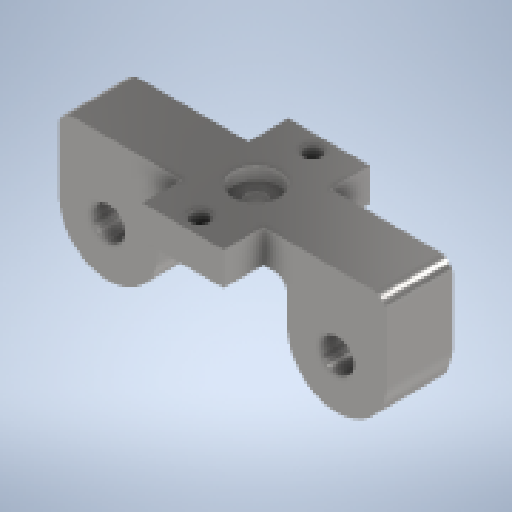
# Autodesk Inventor part: Podstawa chwytaka
Saved by Autodesk Inventor 2024.1 (Build 281209000, 209)
## iProperties
Created: 2024-05-12
Part Number: Podstawa chwytaka
Material: Stal, węglowa
Document SubType Name: Modeling
Designer: Krzysiu
Density: 7.85 g/cm^3
Appearance: Częściowo polerowany
Stock Number: 01
Mass: 49.8719 g
Surface Area: 34.4845 cm^2
Volume: 6.35311 cm^3
Author: Krzysiu
Autodesk Inventor part; units mm, degrees
ref_plane "YZ Plane" through (0, 0, 0) normal (1, 0, 0) x (0, 1, 0)
ref_plane "XZ Plane" through (0, 0, 0) normal (0, 1, 0) x (-1, 0, 0)
ref_plane "XY Plane" through (0, 0, 0) normal (0, 0, 1) x (1, 0, 0)
sketch "Szkic1" plane through (0, 0, 0) normal (0, 0, 1) x (1, 0, 0)
  line L0 (-2.5, 0) -> (-27.5, 0)
  line L1 (-27.5, 0) -> (-19.7354, -28.9778)
  line L2 (-27.5, 0) -> (2.5, 0) construction
  line L3 (-27.5, 0) -> (-37.3351, 36.7052)
  line L4 (-27.5, 0) -> (10.5, 0) construction
  line L5 (-37.3351, 36.7052) -> (-37.3351, 54.7052)
  line L6 (-37.3351, 54.7052) -> (-2.5, 54.7052)
  line L7 (-37.3351, 54.7052) -> (-27.3351, 72.0257)
  line L8 (-37.3351, 54.7052) -> (-17.3351, 54.7052) construction
  line L9 (-37.3351, 54.7052) -> (-27.3351, 37.3847)
  line L10 (-37.3351, 54.7052) -> (-17.3351, 54.7052) construction
  circle A0 centre (-27.5, 0) radius 1.5
  line L11 (-2.5, 0) -> (-2.5, -12)
  line L12 (-2.5, -12) -> (-27.5, -12)
  line L13 (-27.5, -12) -> (-19.7354, -28.9778)
  line L14 (-27.5, -12) -> (-48.0171, 32.862)
  line L15 (-48.0171, 32.862) -> (-51.0127, 50.611)
  line L16 (-48.0171, 32.862) -> (-30.0171, 32.862) construction
  line L17 (-51.0127, 50.611) -> (-38.2696, 35.1962)
  line L18 (-51.0127, 50.611) -> (-31.0127, 50.611) construction
  line L19 (-51.0127, 50.611) -> (-44.0347, 69.3542)
  line L20 (-51.0127, 50.611) -> (-31.0127, 50.611) construction
  circle A1 centre (-27.5, -12) radius 1.5
  line L21 (-19.7354, -28.9778) -> (0, -28.9778)
  circle A2 centre (-19.7354, -28.9778) radius 2.5
  line L22 (-22.2354, -28.9778) -> (-27.2354, -28.9778)
  line L23 (17.2354, -28.9778) -> (22.2354, -28.9778)
  circle A3 centre (14.7354, -28.9778) radius 2.5
  line L24 (22.5, -12) -> (14.7354, -28.9778)
  line L25 (14.7354, -28.9778) -> (0, -28.9778)
  line L26 (-2.5, -12) -> (22.5, -12)
  line L27 (32.3351, 54.7052) -> (22.3351, 37.3847)
  line L28 (32.3351, 36.7052) -> (32.3351, 54.7052)
  line L29 (46.0127, 50.611) -> (33.2696, 35.1962)
  line L30 (43.0171, 32.862) -> (46.0127, 50.611)
  line L31 (43.0171, 32.862) -> (25.0171, 32.862) construction
  circle A4 centre (22.5, 0) radius 1.5
  line L32 (22.5, 0) -> (32.3351, 36.7052)
  circle A5 centre (22.5, -12) radius 1.5
  line L33 (22.5, -12) -> (43.0171, 32.862)
  line L34 (-2.5, 0) -> (22.5, 0)
  line L35 (22.5, 0) -> (14.7354, -28.9778)
  line L36 (22.5, 0) -> (-7.5, 0) construction
  line L37 (22.5, 0) -> (-15.5, 0) construction
  line L38 (46.0127, 50.611) -> (26.0127, 50.611) construction
  line L39 (46.0127, 50.611) -> (26.0127, 50.611) construction
  line L40 (32.3351, 54.7052) -> (12.3351, 54.7052) construction
  line L41 (32.3351, 54.7052) -> (12.3351, 54.7052) construction
  line L42 (32.3351, 54.7052) -> (-2.5, 54.7052)
  line L43 (46.0127, 50.611) -> (39.0347, 69.3542)
  line L44 (32.3351, 54.7052) -> (22.3351, 72.0257)
  line L45 (-19.7354, -31.4778) -> (-19.7354, -36.4778)
  line L46 (-19.7354, -36.4778) -> (0, -36.4778)
  line L47 (-19.7354, -36.4778) -> (-22.2354, -36.4778)
  line L48 (-27.2354, -28.9778) -> (-27.2354, -31.4778)
  line L49 (-19.7354, -26.4778) -> (-19.7354, -21.4778)
  line L50 (-19.7354, -21.4778) -> (-22.2354, -21.4778)
  line L51 (-27.2354, -26.4778) -> (-27.2354, -28.9778)
  line L52 (-19.7354, -21.4778) -> (0, -21.4778)
  line L53 (22.5, 0) -> (14.7354, -28.9778)
  line L54 (22.5, -12) -> (14.7354, -28.9778)
  line L55 (14.7354, -28.9778) -> (-5, -28.9778)
  circle A6 centre (14.7354, -28.9778) radius 2.5
  line L56 (17.2354, -28.9778) -> (22.2354, -28.9778)
  line L57 (-19.7354, -28.9778) -> (-5, -28.9778)
  line L58 (14.7354, -31.4778) -> (14.7354, -36.4778)
  line L59 (14.7354, -36.4778) -> (-5, -36.4778)
  line L60 (14.7354, -36.4778) -> (17.2354, -36.4778)
  line L61 (22.2354, -28.9778) -> (22.2354, -31.4778)
  line L62 (14.7354, -26.4778) -> (14.7354, -21.4778)
  line L63 (14.7354, -21.4778) -> (17.2354, -21.4778)
  line L64 (22.2354, -26.4778) -> (22.2354, -28.9778)
  line L65 (14.7354, -21.4778) -> (-5, -21.4778)
  arc A7 (-22.2354, -21.4778) -> (-27.2354, -26.4778) centre (-22.2354, -26.4778) ccw
  arc A8 (-27.2354, -31.4778) -> (-22.2354, -36.4778) centre (-22.2354, -31.4778) ccw
  arc A9 (22.2354, -26.4778) -> (17.2354, -21.4778) centre (17.2354, -26.4778) ccw
  arc A10 (17.2354, -36.4778) -> (22.2354, -31.4778) centre (17.2354, -31.4778) ccw
  point P0 (0, 0)
  point P1 (-27.2354, -36.4778)
  point P2 (-27.2354, -21.4778)
  point P3 (22.2354, -36.4778)
  point P4 (22.2354, -21.4778)
  dimension "d0" = 25
  dimension "d1" = 30
  dimension "d2" = 75
  dimension "d3" = 38
  dimension "d4" = 105
  dimension "d5" = 18
  dimension "d6" = 20
  dimension "d7" = 60
  dimension "d8" = 20
  dimension "d9" = 60
  dimension "d10" = 3
  dimension "d11" = 12
  dimension "d12" = 25
  dimension "d13" = 49.331
  dimension "d14" = 18
  dimension "d15" = 99.58
  dimension "d16" = 20
  dimension "d17" = 50.42
  dimension "d18" = 20
  dimension "d19" = 69.58
  dimension "d20" = 3
  dimension "d22" = 5
  dimension "d23" = 5
  dimension "d28" = 5
  dimension "d29" = 5
  dimension "d30" = 5
  dimension "d31" = 5
  dimension "d32" = 5
  dimension "d33" = 5
  constraints: 132 end point, 37 symmetric about line, 14 point on circle, 12 horizontal, 12 point on line, 10 centre point, 10 coincident, 8 tangent, 7 equal length, 7 perpendicular, 2 vertical, 1 horizontal alignment, 6 other
  measures "d0" distance of L0.start L0.end
  measures "d1" distance of L0.end L1.end
  measures "d2" angle of L1 L2
  measures "d3" distance of L0.end L3.end
  measures "d4" angle of L4 L3
  measures "d5" distance of L3.end L5.end
  measures "d6" distance of L5.end L7.end
  measures "d7" angle of L8 L7
  measures "d8" distance of L5.end L9.end
  measures "d9" angle of L9 L10
  measures "d10" diameter of A0
  measures "d11" distance of L0.start L11.end
  measures "d12" distance of L11.end L12.end
  measures "d13" distance of L12.end L14.end
  measures "d14" distance of L14.end L15.end
  measures "d15" angle of L16 L15
  measures "d16" distance of L15.end L17.end
  measures "d17" angle of L17 L18
  measures "d18" distance of L15.end L19.end
  measures "d19" angle of L20 L19
  measures "d20" diameter of A1
  measures "d22" diameter of A2
  measures "d23" distance of L22.start L22.end
  measures "d28" distance of L45.start L45.end
  measures "d29" distance of L49.start L49.end
  measures "d30" radius of A7
  measures "d31" radius of A8
  measures "d32" radius of A9
  measures "d33" radius of A10
extrude "Wyciągnięcie proste1" add sketch "Szkic1" along normal mid plane 10 contours L50 L49 A2 L1 | L1 A2 L13 A7 L50 | L63 A9 L24 A3 L35 | L35 A3 L62 L63 | L52 L65 L62 A3 L25 L21 A2 L49 | A2 L22 L51 A7 L13 | A9 L64 L23 A3 L24 | L21 L25 A3 L58 L59 L46 L45 A2 | A2 L45 L47 A8 L48 L22 | L23 L61 A10 L60 L58 A3
sketch "Szkic2" plane through (0, 0, 5) normal (0, 0, 1) x (1, 0, 0)
  circle A0 centre (-19.7354, -28.9778) radius 2.5 projected
  circle A1 centre (-19.7354, -28.9778) radius 2.5
  circle A2 centre (14.7354, -28.9778) radius 2.5 projected
  circle A3 centre (14.7354, -28.9778) radius 2.5
  point P0 (0, 0)
  constraints: 2 centre point, 2 coincident
extrude "Wyciągnięcie proste2" add sketch "Szkic2" along normal blind 10 and the other way blind 20
sketch "Szkic3" plane through (-22.2354, -36.4778, 5) normal (0, -1, 0) x (1, 0, 0)
  line L0 (44.4709, -10) -> (44.4709, 0) projected
  line L1 (44.4709, -5) -> (-5, -5)
  line L2 (-5, -10) -> (-5, 0) projected
  line L3 (0, 0) -> (39.4709, 0) projected
  line L4 (19.7354, 0) -> (19.7354, -10)
  circle A0 centre (19.7354, -5) radius 1.6
  point P0 (22.2354, -5)
  dimension "d40" = 3.2
  constraints: 4 end point, 4 midpoint, 1 centre point, 1 vertical
  measures "d40" diameter of A0
extrude "Wyciągnięcie proste3" cut sketch "Szkic3" against normal through all
sketch "Szkic4" plane through (14.7354, -28.9778, 15) normal (0, 0, 1) x (1, 0, 0)
  circle A0 centre (0, 0) radius 2.5
  circle A1 centre (-34.4709, 0) radius 2.5 projected
  circle A2 centre (-34.4709, 0) radius 2.5
  point P0 (-14.7354, 28.9778)
  constraints: 2 centre point, 1 coincident
extrude "Wyciągnięcie proste4" cut sketch "Szkic4" against normal through all
sketch "Szkic5" plane through (0, 0, 5) normal (0, 0, 1) x (1, 0, 0)
  line L0 (-22.2354, -21.4778) -> (17.2354, -21.4778) projected
  line L1 (0, -21.4778) -> (0, -22.7258)
  line L2 (0, -21.4778) -> (1.248, -21.4778) construction
  circle A0 centre (14.7354, -28.9778) radius 2.5 projected
  circle A1 centre (14.7354, -28.9778) radius 7.5
  circle A2 centre (-19.7354, -28.9778) radius 2.5 projected
  circle A3 centre (-19.7354, -28.9778) radius 7.5
  line L3 (0, -22.7258) -> (7.2354, -22.7258)
  line L4 (7.2354, -22.7258) -> (7.2354, -28.9778)
  line L5 (0, -22.7258) -> (-12.2354, -22.7258)
  line L6 (-12.2354, -22.7258) -> (-12.2354, -28.9778)
  line L7 (22.2354, -28.9778) -> (22.2354, -21.4778)
  line L8 (22.2354, -26.4778) -> (22.2354, -31.4778) projected
  line L9 (7.2354, -22.7258) -> (7.2354, -12.7258)
  line L10 (7.2354, -12.7258) -> (-12.2354, -12.7258)
  line L11 (-12.2354, -12.7258) -> (-27.2354, -12.7258)
  line L12 (-27.2354, -12.7258) -> (-27.2354, -28.9778)
  line L13 (22.2354, -21.4778) -> (22.2354, -12.7258)
  line L14 (22.2354, -12.7258) -> (7.2354, -12.7258)
  line L15 (-27.2354, -12.7258) -> (-27.2354, -17.7258)
  line L16 (-27.2354, -12.7258) -> (-27.2354, -17.7258)
  line L17 (-27.2354, -17.7258) -> (22.2354, -17.7258)
  point P0 (0, 0)
  dimension "d45" = 1.248
  dimension "d46" = 270
  dimension "d47" = 7.5
  dimension "d48" = 10
  constraints: 32 end point, 7 perpendicular, 6 point on line, 4 point on circle, 3 collinear, 2 centre point, 2 coincident, 2 horizontal, 2 tangent, 1 parallel, 1 vertical
  measures "d45" distance of L1.start L1.end
  measures "d47" distance of L7.start L7.end
  measures "d48" distance of L3.end L9.end
extrude "Wyciągnięcie proste5" add sketch "Szkic5" along normal blind 10 contours A3 L12 L17 L9 L0 | L0 L1 L5 L6 A3 | A3 | L0 L9 L3 L1 | L9 L17 L13 L7 A1 L0 | L0 A1 L4 L9 | A1
sketch "Szkic6" plane through (0, 0, -5) normal (0, 0, -1) x (-1, 0, 0)
  line L0 (22.2354, -21.4778) -> (-17.2354, -21.4778) projected
  arc A0 (-17.2354, -21.4778) -> (-22.2354, -26.4778) centre (-17.2354, -26.4778) ccw projected
  line L1 (-22.2354, -26.4778) -> (-22.2354, -31.4778) projected
  arc A1 (-22.2354, -31.4778) -> (-17.2354, -36.4778) centre (-17.2354, -31.4778) ccw projected
  line L2 (-17.2354, -36.4778) -> (22.2354, -36.4778) projected
  arc A2 (22.2354, -36.4778) -> (27.2354, -31.4778) centre (22.2354, -31.4778) ccw projected
  line L3 (27.2354, -31.4778) -> (27.2354, -26.4778) projected
  arc A3 (27.2354, -26.4778) -> (22.2354, -21.4778) centre (22.2354, -26.4778) ccw projected
  point P0 (0, 0)
extrude "Wyciągnięcie proste6" cut sketch "Szkic6" against normal blind 10
fillet "Zaokrąglenie1" radius 2 4 edges at (-12.2354, -22.7258, 10) (7.2354, -22.7258, 10) (22.2354, -17.7258, 10) (-27.2354, -17.7258, 10)
sketch "Szkic7" plane through (-25.2354, -17.7258, 5) normal (0, 1, 0) x (1, 0, 0)
  line L0 (15, -10) -> (30.4709, -10) projected
  line L1 (22.7354, -10) -> (28.8669, -10)
  line L2 (28.8669, -10) -> (28.8669, -16)
  line L3 (28.8669, -16) -> (16.6039, -16)
  line L4 (16.6039, -16) -> (16.6039, -10)
  line L5 (22.7354, -10) -> (16.6039, -10)
  line L6 (16.6039, -10) -> (16.6039, 0)
  line L7 (22.7354, 6) -> (28.8669, 6)
  line L8 (28.8669, 6) -> (28.8669, 0)
  line L9 (28.8669, 0) -> (16.6039, 0)
  line L10 (16.6039, 0) -> (16.6039, 6)
  line L11 (22.7354, 6) -> (16.6039, 6)
  point P0 (25.2354, 5)
  dimension "d54" = 6.1315
  dimension "d55" = 6
  dimension "d56" = 12.263
  dimension "d57" = 10
  dimension "d58" = 6.1315
  dimension "d59" = 6
  dimension "d60" = 12.263
  constraints: 22 end point, 3 perpendicular, 3 vertical, 2 horizontal, 2 point on line, 1 midpoint
  measures "d54" distance of L1.start L1.end
  measures "d55" distance of L1.end L2.end
  measures "d56" distance of L2.end L3.end
  measures "d57" distance of L4.end L6.end
  measures "d58" distance of L7.start L7.end
  measures "d59" distance of L7.end L8.end
  measures "d60" distance of L8.end L9.end
extrude "Wyciągnięcie proste7" add sketch "Szkic7" against normal up to surface (5 mm away)
sketch "Szkic8" plane through (-25.2354, -17.7258, 15) normal (0, 1, 0) x (1, 0, 0)
  line L0 (28.8669, 16) -> (16.6039, 16) projected
  line L1 (22.7354, 16) -> (22.7354, -6)
  line L2 (16.6039, -6) -> (28.8669, -6) projected
  circle A0 centre (22.7354, 5) radius 1.6
  point P0 (25.2354, 15)
  dimension "d64" = 3.2
  constraints: 3 midpoint, 2 end point, 1 centre point
  measures "d64" diameter of A0
extrude "Wyciągnięcie proste8" cut sketch "Szkic8" against normal blind 10
sketch "Szkic9" plane through (-25.2354, -17.7258, 15) normal (0, 1, 0) x (1, 0, 0)
  point P0 (22.7354, 13.5)
hole "Otwór1" at (-2.5, -17.7258, 1.5) direction (0, -1, 0) diameter 2.9 end through all
sketch "Szkic10" plane through (-25.2354, -17.7258, 15) normal (0, 1, 0) x (1, 0, 0)
  point P0 (22.7354, -3.5)
hole "Otwór2" at (-2.5, -17.7258, 18.5) direction (0, -1, 0) diameter 2.9 end through all
sketch "Szkic11" plane through (-25.2354, -17.7258, 15) normal (0, 1, 0) x (1, 0, 0)
  circle A0 centre (22.7354, 5) radius 1.6 projected
  circle A1 centre (22.7354, 5) radius 3.5
  point P0 (25.2354, 15)
  dimension "d81" = 7
  constraints: 1 centre point, 1 coincident
  measures "d81" diameter of A1
extrude "Wyciągnięcie proste9" cut sketch "Szkic11" against normal blind 2
